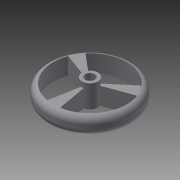
# Autodesk Inventor part: wheel
Saved by Autodesk Inventor 2015 (Build 190159000, 159)
## iProperties
Created: 2014-10-24
Part Number: wheel
Material: Generic
Document SubType Name: Modeling
Designer: Colin
Density: 1 g/cm^3
Appearance: Default
Author: Colin
Autodesk Inventor part; units mm, degrees
ref_plane "YZ Plane" through (0, 0, 0) normal (1, 0, 0) x (0, 1, 0)
ref_plane "XZ Plane" through (0, 0, 0) normal (0, 1, 0) x (-1, 0, 0)
ref_plane "XY Plane" through (0, 0, 0) normal (0, 0, 1) x (1, 0, 0)
sketch "Sketch2" plane through (0, 0, 0) normal (0, 1, 0) x (-1, 0, 0)
  circle A0 centre (0, 0) radius 14
  line L0 (0, 0) -> (0, 14) construction
  line L1 (0, 0) -> (12.1244, -7) construction
  line L2 (0, 0) -> (-12.1244, -7) construction
  circle A1 centre (0, 0) radius 3
  line L3 (2.8191, -1.0261) -> (13.1557, -4.7883)
  line L4 (2.2981, -1.9284) -> (10.7246, -8.999)
  line L5 (0.5209, 2.9544) -> (2.4311, 13.7873)
  line L6 (-0.5209, 2.9544) -> (-2.4311, 13.7873)
  line L7 (-2.8191, -1.0261) -> (-13.1557, -4.7883)
  line L8 (-2.2981, -1.9284) -> (-10.7246, -8.999)
  circle A2 centre (0, 0) radius 16
  circle A3 centre (0, 0) radius 1.8196
  dimension "d10" = 120
  dimension "d11" = 120
  dimension "d18" = 6
  dimension "d19" = 10
  dimension "d20" = 20
  dimension "d21" = 10
  dimension "d22" = 20
  dimension "d23" = 10
  dimension "d24" = 20
  dimension "d26" = 3.6391
  dimension "d29" = 32
  dimension "d30" = 2
  constraints: 18 end point, 6 point on circle, 4 coincident, 3 centre point, 1 vertical, 11 other
  measures "d10" angle of L0 L1
  measures "d11" angle of L0 L2
  measures "d18" diameter of A1
  measures "d19" angle of L1 L3
  measures "d20" angle of L4 L3
  measures "d21" angle of L0 L5
  measures "d22" angle of L6 L5
  measures "d23" angle of L2 L7
  measures "d24" angle of L8 L7
  measures "d26" diameter of A3
  measures "d29" diameter of A2
extrude "Extrusion1" add sketch "Sketch2" along normal blind 6.6 contours L5 A1 L6 A0 | A0 L4 A1 L3 | A1 | L7 A1 L8 A0 | A2
sketch "Sketch3" plane through (0, 6.6, 0) normal (0, 1, 0) x (1, 0, 0)
  circle A0 centre (0, 0) radius 3
  circle A1 centre (0, 0) radius 1.8196 projected
  circle A2 centre (0, 0) radius 1.8196
  constraints: 2 centre point, 2 coincident
extrude "Extrusion2" add sketch "Sketch3" along normal blind 2
fillet "Fillet4" radius 2.54 2 edges at (16, 6.6, 0) (16, 0, 0)
body "Solid1"
